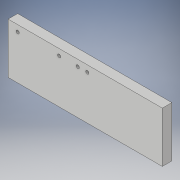
# Autodesk Inventor part: Kermit bumper 2 medium
Saved by Autodesk Inventor 2018.2 (Build 222227000, 227)
## iProperties
Created: 2018-02-13
Part Number: Kermit bumper 2 medium
Material: Generic
Document SubType Name: Modeling
Designer: kalra.rohan
Density: 1 g/cm^3
Appearance: Default
Author: kalra.rohan
Autodesk Inventor part; units mm, degrees
ref_plane "YZ Plane" through (0, 0, 0) normal (1, 0, 0) x (0, 1, 0)
ref_plane "XZ Plane" through (0, 0, 0) normal (0, 1, 0) x (-1, 0, 0)
ref_plane "XY Plane" through (0, 0, 0) normal (0, 0, 1) x (1, 0, 0)
sketch "Sketch1" plane through (0, 0, 0) normal (0, 0, 1) x (1, 0, 0)
  line L0 (0, 0) -> (368.3, 0)
  line L1 (368.3, 0) -> (368.3, -120.65)
  line L2 (368.3, -120.65) -> (0, -120.65)
  line L3 (0, -120.65) -> (0, 0)
  circle A0 centre (22.86, -15.24) radius 3.81
  circle A1 centre (121.92, -15.24) radius 3.81
  circle A2 centre (166.37, -15.24) radius 3.81
  circle A3 centre (189.23, -15.24) radius 3.81
  dimension "d0" = 368.3
  dimension "d1" = 120.65
  dimension "d2" = 7.62
  dimension "d3" = 22.86
  dimension "d4" = 105.41
  dimension "d5" = 7.62
  dimension "d6" = 99.06
  dimension "d7" = 7.62
  dimension "d8" = 44.45
  dimension "d9" = 7.62
  dimension "d10" = 22.86
  constraints: 8 end point, 4 centre point, 2 parallel, 1 horizontal, 1 perpendicular
  measures "d0" distance between parallel lines of L1 L3
  measures "d1" distance between parallel lines of L0 L2
  measures "d2" diameter of A0
  measures "d3" distance from line of L3 A0.centre
  measures "d4" distance from line of A0.centre L2
  measures "d5" diameter of A1
  measures "d6" distance of A1.centre A0.centre
  measures "d7" diameter of A2
  measures "d8" distance of A2.centre A1.centre
  measures "d9" diameter of A3
  measures "d10" distance of A3.centre A2.centre
extrude "Extrusion1" add sketch "Sketch1" against normal blind 22.86
body "Solid1"
